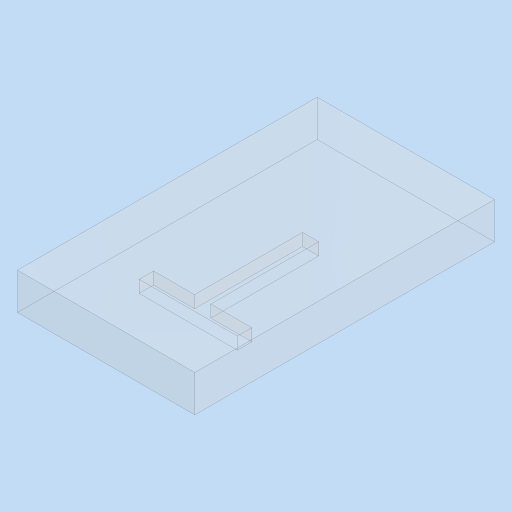
# Autodesk Inventor part: pegshort
Saved by Autodesk Inventor 2023 (Build 270158000, 158)
## iProperties
Created: 2026-03-30
Part Number: pegshort
Material: PET Plastic
Document SubType Name: Modeling
Designer: Nathann
Density: 1.541 g/cm^3
Appearance: Polycarbonate - Clear
Author: Nathann
Autodesk Inventor part; units mm, degrees
ref_plane "YZ Plane" through (0, 0, 0) normal (1, 0, 0) x (0, 1, 0)
ref_plane "XZ Plane" through (0, 0, 0) normal (0, 1, 0) x (-1, 0, 0)
ref_plane "XY Plane" through (0, 0, 0) normal (0, 0, 1) x (1, 0, 0)
sketch "Sketch1" plane through (0, 0, 0) normal (0, 1, 0) x (-1, 0, 0)
  line L0 (0, 0) -> (29, 0)
  line L1 (29, 0) -> (29, 49)
  line L2 (29, 49) -> (0, 49)
  line L3 (0, 49) -> (0, 0)
  dimension "d0" = 49
  dimension "d1" = 29
  constraints: 8 end point, 2 parallel, 1 horizontal, 1 perpendicular
  measures "d0" distance of L0.end L1.end
  measures "d1" distance of L1.end L2.end
extrude "Extrusion1" add sketch "Sketch1" along normal blind 6
sketch "Sketch2" plane through (0, 0, 0) normal (0, -1, 0) x (1, 0, 0)
  line L0 (-21.7451, 36.3583) -> (64.7541, 36.3583) construction
  line L1 (64.7541, 36.3583) -> (64.7541, 15.5155) construction
  line L2 (64.7541, 15.5155) -> (-21.7451, 15.5155) construction
  line L3 (-21.7451, 15.5155) -> (-21.7451, 36.3583) construction
  line L4 (-15.0514, 16.3583) -> (-15.0514, 33.992)
  line L5 (-15.0514, 33.992) -> (-21.7613, 33.992)
  line L6 (-21.7613, 33.992) -> (-21.7613, 36.3583)
  line L7 (-21.7613, 36.3583) -> (-5.6835, 36.3583)
  line L8 (-5.6835, 36.3583) -> (-5.6835, 33.992)
  line L9 (-5.6835, 33.992) -> (-12.3934, 33.992)
  line L10 (-12.3934, 33.992) -> (-12.3934, 16.3583)
  line L11 (-12.3934, 16.3583) -> (-15.0514, 16.3583)
  point P0 (0, 0)
  constraints: 2 other
emboss "Emboss1" sketch "Sketch2" operation cut depth 2 direction (0, 1, 0)
body "Solid1"
